# Autodesk Inventor part: D0-D3_1X04_NO_SILK_ALL_ROUND
Saved by Autodesk Inventor 2016 (Build 200138000, 138)
## iProperties
Created: 2016-04-08
Part Number: D0-D3_1X04_NO_SILK_ALL_ROUND
Material: Generic
Document SubType Name: Modeling
Designer: Paschalis
Density: 1 g/cm^3
Appearance: 1X04_NO_SILK_ALL_ROUND, D0-D3_1X04_NO_SILK_ALL_ROUND
Author: Paschalis
Autodesk Inventor part; units mm, degrees
ref_plane "YZ Plane" through (0, 0, 0) normal (1, 0, 0) x (0, 1, 0)
ref_plane "XZ Plane" through (0, 0, 0) normal (0, 1, 0) x (-1, 0, 0)
ref_plane "XY Plane" through (0, 0, 0) normal (0, 0, 1) x (1, 0, 0)
sketch "1X04_NO_SILK_ALL_ROUND, D0-D3_1X04_NO_SILK_ALL_ROUND_59" plane through (0, 0, 0) normal (0, 0, 1) x (1, 0, 0)
  line L0 (-0.254, 0.254) -> (7.874, 0.254)
  line L1 (7.874, 0.254) -> (7.874, -0.254)
  line L2 (7.874, -0.254) -> (-0.254, -0.254)
  line L3 (-0.254, -0.254) -> (-0.254, 0.254)
  constraints: 8 end point
extrude "Extrusion1" add sketch "1X04_NO_SILK_ALL_ROUND, D0-D3_1X04_NO_SILK_ALL_ROUND_59" along normal blind 1
body "Solid1"
